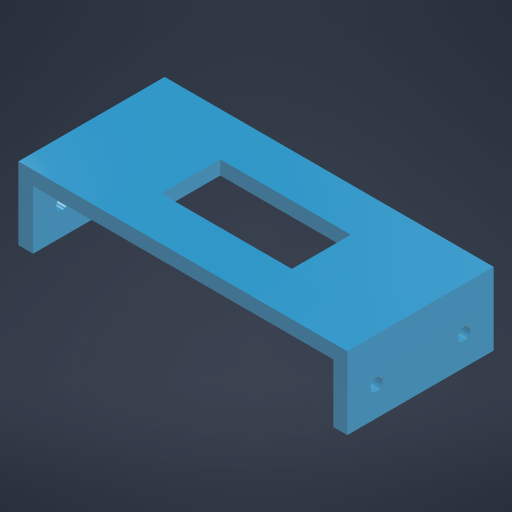
# Autodesk Inventor part: Power Switch Mount
Saved by Autodesk Inventor 2024.2 (Build 282272000, 272)
## iProperties
Created: 2024-01-11
Part Number: Power Switch Mount
Material: Generic
Document SubType Name: Modeling
Designer: student
Density: 1 g/cm^3
Appearance: Default
Author: student
Autodesk Inventor part; units mm, degrees
ref_plane "YZ Plane" through (0, 0, 0) normal (1, 0, 0) x (0, 1, 0)
ref_plane "XZ Plane" through (0, 0, 0) normal (0, 1, 0) x (-1, 0, 0)
ref_plane "XY Plane" through (0, 0, 0) normal (0, 0, 1) x (1, 0, 0)
sketch "Sketch1" plane through (0, 0, 0) normal (0, 1, 0) x (-1, 0, 0)
  line L0 (0, 0) -> (71.374, 0)
  line L1 (71.374, 0) -> (71.374, -19.05)
  line L2 (0, -19.05) -> (0, 0)
  line L3 (71.374, -19.05) -> (71.374, -31.75)
  line L4 (71.374, -31.75) -> (0, -31.75)
  line L5 (0, -31.75) -> (0, -19.05)
  line L6 (71.374, 0) -> (71.374, -6.35)
  line L7 (71.374, -6.35) -> (87.352, -6.35)
  line L8 (71.374, -31.75) -> (71.374, -25.4)
  line L9 (71.374, -25.4) -> (87.352, -25.4)
  line L10 (71.374, -6.35) -> (-10.213, -6.35)
  line L11 (71.374, -25.4) -> (-10.213, -25.4)
  dimension "d0" = 71.374
  dimension "d1" = 19.05
  dimension "d2" = 12.7
  dimension "d3" = 6.35
  dimension "d4" = 6.35
  constraints: 24 end point, 6 perpendicular, 2 horizontal, 1 midpoint, 1 point on line, 1 vertical
  measures "d0" distance of L0.start L0.end
  measures "d1" distance of L0.end L1.end
  measures "d2" distance of L1.end L3.end
  measures "d3" distance of L0.end L6.end
  measures "d4" distance of L3.end L8.end
extrude "Extrusion1" add sketch "Sketch1" along normal blind 3.048
sketch "Sketch2" plane through (0, 3.048, 0) normal (0, 1, 0) x (1, 0, 0)
  line L0 (-71.374, 0) -> (0, 0) projected
  line L1 (0, 0) -> (0, 6.35)
  line L2 (0, 0) -> (0, 31.75) projected
  line L3 (0, 6.35) -> (-71.374, 6.35)
  line L4 (-71.374, 31.75) -> (-71.374, 0) projected
  line L5 (-71.374, 31.75) -> (-71.374, 25.4)
  line L6 (-71.374, 25.4) -> (0, 25.4)
  line L7 (0, 6.35) -> (0, 10.7315)
  line L8 (0, 10.7315) -> (-19.0957, 10.7315)
  line L9 (0, 25.4) -> (0, 21.0185)
  line L10 (0, 21.0185) -> (-20.1254, 21.0185)
  line L11 (0, 10.7315) -> (-22.7876, 10.7315)
  line L12 (-71.374, 6.35) -> (-71.374, 10.7315)
  line L13 (-71.374, 10.7315) -> (-48.5864, 10.7315)
  line L14 (-48.5864, 10.7315) -> (-48.5864, 21.0185)
  line L15 (-48.5864, 21.0185) -> (-71.374, 21.0185)
  line L16 (-22.7876, 10.7315) -> (-22.7876, 21.0185)
  line L17 (-22.7876, 21.0185) -> (-20.1254, 21.0185)
  line L18 (-22.7876, 10.7315) -> (-48.5864, 10.7315)
  line L19 (-48.5864, 21.0185) -> (-22.7876, 21.0185)
  line L20 (-21.5176, 10.7315) -> (-21.5176, 21.0185)
  line L21 (-49.8564, 10.7315) -> (-49.8564, 21.0185)
  line L22 (-22.7876, 9.4615) -> (-48.5864, 9.4615)
  line L23 (-48.5864, 22.2885) -> (-22.7876, 22.2885)
  line L24 (-48.5864, 9.4615) -> (-49.8564, 9.4615)
  line L25 (-49.8564, 9.4615) -> (-49.8564, 10.7315)
  line L26 (-49.8564, 21.0185) -> (-49.8564, 22.2885)
  line L27 (-49.8564, 22.2885) -> (-48.5864, 22.2885)
  line L28 (-22.7876, 22.2885) -> (-21.5176, 22.2885)
  line L29 (-21.5176, 22.2885) -> (-21.5176, 21.0185)
  line L30 (-21.5176, 10.7315) -> (-21.5176, 9.4615)
  line L31 (-22.7876, 9.4615) -> (-21.5176, 9.4615)
  dimension "d7" = 6.35
  dimension "d8" = 6.35
  dimension "d9" = 4.3815
  dimension "d10" = 4.3815
  dimension "d11" = 22.7876
  dimension "d12" = 4.3815
  dimension "d13" = 22.7876
  dimension "d14" = 1.27
  dimension "d15" = 1.27
  dimension "d16" = 1.27
  dimension "d17" = 1.27
  constraints: 58 end point, 12 point on line, 11 perpendicular, 5 parallel, 2 horizontal, 1 vertical
  measures "d7" distance of L0.end L1.end
  measures "d8" distance of L4.start L5.end
  measures "d9" distance of L1.end L7.end
  measures "d10" distance of L6.end L9.end
  measures "d11" distance of L7.end L11.end
  measures "d12" distance of L3.end L12.end
  measures "d13" distance of L12.end L13.end
  measures "d14" distance between parallel lines of L16 L20
  measures "d15" distance between parallel lines of L14 L21
  measures "d16" distance between parallel lines of L18 L22
  measures "d17" distance between parallel lines of L19 L23
extrude "Extrusion2" cut sketch "Sketch2" against normal blind 19.177 contours L21 L15 L14 L13 | L13 L18 L11 L30 L31 L22 L24 L25 | L26 L27 L23 L28 L29 L17 L19 L15 | L14 L19 L16 L18 | L11 L16 L17 L20
sketch "Sketch3" plane through (0, 0, 0) normal (0, -1, 0) x (1, 0, 0)
  line L0 (0, -31.75) -> (-71.374, -31.75) projected
  line L1 (0, -31.75) -> (-3.048, -31.75)
  line L2 (-3.048, -31.75) -> (-3.048, 0)
  line L3 (-3.048, 0) -> (0, 0)
  line L4 (0, 0) -> (0, -31.75) projected
  line L5 (0, 0) -> (0, -31.75)
  line L6 (-71.374, -31.75) -> (-68.1711, -31.75)
  line L7 (-68.1711, -31.75) -> (-68.1711, 0)
  line L8 (-71.374, 0) -> (0, 0) projected
  line L9 (-71.374, 0) -> (-68.1711, 0)
  line L10 (-71.374, 0) -> (-71.374, -31.75)
  dimension "d20" = 3.048
  constraints: 16 end point, 4 perpendicular, 3 point on line, 2 collinear
  measures "d20" distance of L0.start L1.end
extrude "Extrusion3" add sketch "Sketch3" along normal blind 12.7 contours L0 L2 L3 L4 | L0 L10 L8 L7
sketch "Sketch4" plane through (0, 3.048, 0) normal (1, 0, 0) x (0, 0, -1)
  line L0 (0, -15.748) -> (0, 0) projected
  line L1 (0, 0) -> (0, -15.748)
  line L2 (0, -15.748) -> (0, -3.048)
  line L3 (0, -3.048) -> (31.75, -3.048) projected
  line L4 (0, -3.048) -> (31.75, -3.048)
  line L5 (31.75, -3.048) -> (31.75, -15.748)
  line L6 (31.75, -15.748) -> (0, -15.748)
  line L7 (0, -15.748) -> (0, -10.7569)
  line L8 (0, -10.7569) -> (31.75, -10.7569)
  line L9 (0, -3.048) -> (0, -8.0429)
  line L10 (0, -8.0429) -> (31.75, -8.0429)
  line L11 (0, -10.7569) -> (0, -9.398)
  line L12 (0, -9.398) -> (6.35, -9.398)
  circle A0 centre (6.35, -9.398) radius 1.3551
  line L13 (31.75, -9.398) -> (25.4, -9.398)
  circle A1 centre (25.4, -9.398) radius 1.3551
  dimension "d23" = 12.7
  dimension "d24" = 4.9911
  dimension "d25" = 4.9949
  dimension "d26" = 31.75
  dimension "d27" = 1.3589
  dimension "d28" = 6.35
  dimension "d29" = 6.35
  constraints: 24 end point, 6 perpendicular, 4 point on line, 2 centre point, 2 coincident, 2 collinear, 2 midpoint, 2 tangent, 1 horizontal
  measures "d23" distance of L0.start L2.end
  measures "d24" distance of L0.start L7.end
  measures "d25" distance of L2.end L9.end
  measures "d26" distance of L2.end L3.end
  measures "d27" distance of L7.end L11.end
  measures "d28" distance of L11.end L12.end
  measures "d29" distance of L13.start L13.end
extrude "Extrusion4" cut sketch "Sketch4" against normal blind 96.8375 contours A0 | A1
body "Solid1"
